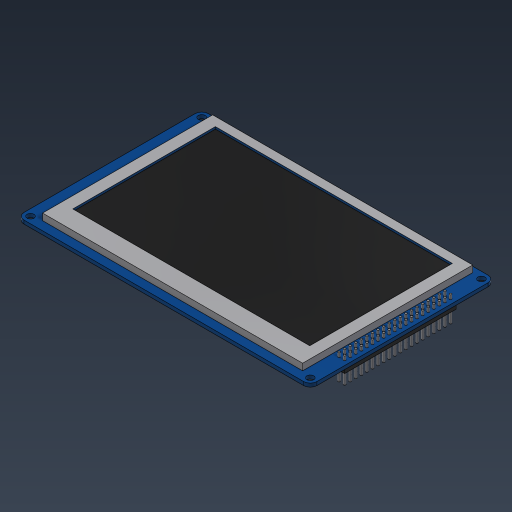
# Autodesk Inventor part: TFT-CP11009
Saved by Autodesk Inventor 2023.1 (Build 271208000, 208)
## iProperties
Created: 2017-10-12
Part Number: TFT-CP11009
Material: Phenolharz
Document SubType Name: Modeling
Designer: ryll
Density: 1.38 g/cm^3
Appearance: Glatt - hellorange
Mass: 53.0055 g
Surface Area: 246.223 cm^2
Volume: 38.4098 cm^3
Author: ryll
Autodesk Inventor part; units mm, degrees
ref_plane "YZ Plane" through (0, 0, 0) normal (1, 0, 0) x (0, 1, 0)
ref_plane "XZ Plane" through (0, 0, 0) normal (0, 1, 0) x (-1, 0, 0)
ref_plane "XY Plane" through (0, 0, 0) normal (0, 0, 1) x (1, 0, 0)
sketch "Skizze1" plane through (0, 0, 0) normal (0, 0, 1) x (1, 0, 0)
  line L0 (-66.75, -42) -> (66.75, -42)
  line L1 (66.75, -42) -> (66.75, 42)
  line L2 (66.75, 42) -> (-66.75, 42)
  line L3 (-66.75, 42) -> (-66.75, -42)
  line L4 (-66.75, -42) -> (66.75, 42) construction
  line L5 (66.75, -42) -> (-66.75, 42) construction
  point P0 (0, 0)
  dimension "d0" = 133.5
  dimension "d1" = 84
  constraints: 12 end point, 2 midpoint, 2 parallel, 1 horizontal, 1 perpendicular
  measures "d0" distance of L2.end L1.end
  measures "d1" distance of L1.end L0.end
extrude "Extrusion1" add sketch "Skizze1" along normal blind 1.6
sketch "Skizze2" plane through (0, 0, 1.6) normal (0, 0, 1) x (1, 0, 0)
  line L0 (-66.75, -42) -> (66.75, -42) projected
  line L1 (66.75, -42) -> (66.75, 42) projected
  line L2 (66.75, 42) -> (-66.75, 42) projected
  line L3 (-66.75, 42) -> (-66.75, -42) projected
  line L4 (-63.75, 39) -> (63.75, 39)
  line L5 (63.75, 39) -> (63.75, -39)
  line L6 (63.75, -39) -> (-63.75, -39)
  line L7 (-63.75, -39) -> (-63.75, 39)
  point P0 (0, 0)
  dimension "d4" = 3
  constraints: 8 end point, 4 coincident, 3 other
  measures "d4" distance between parallel lines of L2 L4
hole "Bohrung1" at (-63.75, 39, 1.6) at (63.75, 39, 1.6) at (-63.75, -39, 1.6) at (63.75, -39, 1.6) direction (0, 0, -1) diameter 3.2 end through all
sketch "Skizze3" plane through (0, 0, 1.6) normal (0, 0, 1) x (1, 0, 0)
  line L0 (-59.25, -38) -> (59.25, -38)
  line L1 (59.25, -38) -> (59.25, 39.5)
  line L2 (59.25, 39.5) -> (-59.25, 39.5)
  line L3 (-59.25, 39.5) -> (-59.25, -38)
  line L4 (-66.75, 42) -> (-66.75, -42) projected
  line L5 (66.75, 42) -> (-66.75, 42) projected
  point P0 (0, 0)
  dimension "d12" = 118.5
  dimension "d13" = 77.5
  dimension "d14" = 7.5
  dimension "d15" = 2.5
  constraints: 8 end point, 2 parallel, 1 horizontal, 1 perpendicular
  measures "d12" distance of L2.end L1.end
  measures "d13" distance of L1.end L0.end
  measures "d14" distance between parallel lines of L4 L3
  measures "d15" distance between parallel lines of L5 L2
extrude "Extrusion2" add sketch "Skizze3" along normal blind 3
sketch "Skizze4" plane through (0, 0, 4.6) normal (0, 0, 1) x (1, 0, 0)
  line L0 (-54, -29.5) -> (54, -29.5)
  line L1 (54, -29.5) -> (54, 35.5)
  line L2 (54, 35.5) -> (-54, 35.5)
  line L3 (-54, 35.5) -> (-54, -29.5)
  line L4 (-59.25, -38) -> (59.25, -38) projected
  line L5 (59.25, -38) -> (59.25, 39.5) projected
  line L6 (59.25, 39.5) -> (-59.25, 39.5) projected
  line L7 (-59.25, 39.5) -> (-59.25, -38) projected
  line L8 (-59.25, 39.5) -> (59.25, 39.5) construction
  line L9 (0, 39.5) -> (0, -38) construction
  point P0 (0, 0)
  dimension "d18" = 108
  dimension "d19" = 65
  dimension "d20" = 4
  constraints: 10 end point, 2 midpoint, 2 parallel, 1 horizontal, 1 perpendicular, 1 other
  measures "d18" distance of L1.end L2.end
  measures "d19" distance of L0.end L1.end
  measures "d20" distance between parallel lines of L6 L2
extrude "Extrusion3" cut sketch "Skizze4" against normal blind 1 contours L3 L2 L1 L0
fillet "Rundung1" radius 3 4 edges at (-66.75, -42, 0.8) (66.75, -42, 0.8) (66.75, 42, 0.8) (-66.75, 42, 0.8)
sketch "Skizze5" plane through (0, 0, 0) normal (0, 0, -1) x (-1, 0, 0)
  line L0 (-60.71, -25.4) -> (-65.79, -25.4)
  line L1 (-65.79, -25.4) -> (-65.79, 25.4)
  line L2 (-65.79, 25.4) -> (-60.71, 25.4)
  line L3 (-60.71, 25.4) -> (-60.71, -25.4)
  line L4 (-93.45, 0) -> (93.45, 0) projected
  arc A0 (66.75, 39) -> (63.75, 42) centre (63.75, 39) ccw projected
  line L5 (-63.75, 42) -> (63.75, 42) projected
  arc A1 (-63.75, 42) -> (-66.75, 39) centre (-63.75, 39) ccw projected
  line L6 (-66.75, -39) -> (-66.75, 39) projected
  arc A2 (-66.75, -39) -> (-63.75, -42) centre (-63.75, -39) ccw projected
  line L7 (63.75, -42) -> (-63.75, -42) projected
  arc A3 (63.75, -42) -> (66.75, -39) centre (63.75, -39) ccw projected
  line L8 (66.75, 39) -> (66.75, -39) projected
  circle A4 centre (63.75, -39) radius 1.6 projected
  circle A5 centre (63.75, 39) radius 1.6 projected
  circle A6 centre (-63.75, 39) radius 1.6 projected
  circle A7 centre (-63.75, -39) radius 1.6 projected
  point P0 (0, 0)
  dimension "d24" = 50.8
  dimension "d25" = 5.08
  dimension "d26" = 0.96
  constraints: 8 end point, 2 parallel, 1 horizontal, 1 perpendicular, 1 other
  measures "d24" distance of L0.end L1.end
  measures "d25" distance of L0.start L0.end
  measures "d26" distance between parallel lines of L6 L1
extrude "Extrusion4" add sketch "Skizze5" along normal blind 2.54 contours L0 L1 L4 L3 | L4 L1 L2 L3
sketch "Skizze6" plane through (0, 0, -2.54) normal (0, 0, -1) x (-1, 0, 0)
  line L0 (-65.79, -25.4) -> (-60.71, -25.4) projected
  line L1 (-60.71, -25.4) -> (-60.71, 25.4) projected
  line L2 (-60.71, 25.4) -> (-65.79, 25.4) projected
  line L3 (-65.79, 25.4) -> (-65.79, -25.4) projected
  circle A0 centre (-61.98, 24.13) radius 0.5
  point P0 (0, 0)
  dimension "d29" = 1
  dimension "d30" = 1.27
  dimension "d31" = 1.27
  constraints: 1 centre point
  measures "d29" diameter of A0
  measures "d30" distance from line of A0.centre L2
  measures "d31" distance from line of L1 A0.centre
extrude "Extrusion5" add sketch "Skizze6" along normal blind 5.5 and the other way blind 6 contours A0
pattern_linear "Rechteckige Anordnung1" count 20 spacing 2.54 along (0, -1, 0) count 2 spacing 2.54 along (1, 0, 0) of "Extrusion5"
